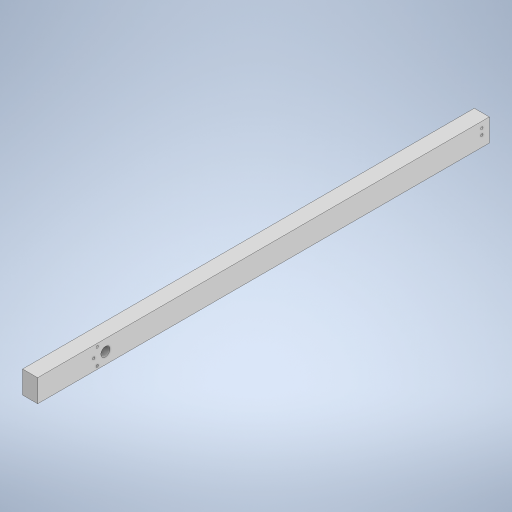
# Autodesk Inventor part: 射出_腕_真
Saved by Autodesk Inventor 2023 (Build 270158000, 158)
## iProperties
Created: 2022-04-27
Part Number: 射出_腕_真
Material: 一般
Document SubType Name: Modeling
Designer: yuta
Density: 1 g/cm^3
Appearance: 既定
Author: yuta
Autodesk Inventor part; units mm, degrees
ref_plane "YZ Plane" through (0, 0, 0) normal (1, 0, 0) x (0, 1, 0)
ref_plane "XZ Plane" through (0, 0, 0) normal (0, 1, 0) x (-1, 0, 0)
ref_plane "XY Plane" through (0, 0, 0) normal (0, 0, 1) x (1, 0, 0)
sketch "スケッチ1" plane through (0, 0, 0) normal (0, 0, 1) x (1, 0, 0)
  line L0 (0, 0) -> (20, 0)
  line L1 (20, 0) -> (20, 30)
  line L2 (20, 30) -> (0, 30)
  line L3 (0, 30) -> (0, 0)
  dimension "d0" = 20
  dimension "d1" = 30
  constraints: 8 end point, 2 parallel, 1 horizontal, 1 perpendicular
  measures "d0" distance of L2.end L1.end
  measures "d1" distance of L1.end L0.end
extrude "押し出し1" add sketch "スケッチ1" along normal blind 600
sketch "スケッチ2" plane through (20, 0, 0) normal (1, 0, 0) x (0, 0, -1)
  circle A0 centre (-510, 15) radius 6.05
  line L0 (0, 30) -> (-600, 30) projected
  line L1 (-600, 0) -> (-600, 30) projected
  point P0 (0, 0)
  dimension "d4" = 12.1
  dimension "d5" = 15
  dimension "d6" = 90
  constraints: 1 centre point
  measures "d4" diameter of A0
  measures "d5" distance from line of L0 A0.centre
  measures "d6" distance from line of L1 A0.centre
extrude "押し出し2" cut sketch "スケッチ2" against normal blind 600
sketch "スケッチ3" plane through (20, 0, 0) normal (1, 0, 0) x (0, 0, -1)
  line L0 (0, 30) -> (-600, 30) projected
  line L1 (0, 0) -> (0, 30) projected
  point P0 (-10, 22)
  point P1 (-10, 14)
  dimension "d9" = 8
  dimension "d10" = 10
  dimension "d11" = 8
  dimension "d12" = 10
  measures "d9" distance from line of L0 point (-10, 22)
  measures "d10" distance from line of L1 point (-10, 22)
  measures "d11" distance of point (-10, 22) point (-10, 14)
  measures "d12" distance from line of L1 point (-10, 14)
hole "穴1" at (20, 22, 10) at (20, 14, 10) direction (-1, 0, 0) diameter 3.2 end through all
sketch "スケッチ4" plane through (20, 0, 0) normal (1, 0, 0) x (0, 0, -1)
  circle A0 centre (-510, 15) radius 6.05 projected
  circle A1 centre (-510, 15) radius 15.5 construction
  line L0 (-510, 15) -> (-527.6598, 32.6598) construction
  line L1 (-510, 15) -> (-485.0253, 15) construction
  line L2 (-527.6598, 32.6598) -> (-527.6598, -10.8806) construction
  line L3 (0, 0) -> (-600, 0) projected
  line L4 (-510, 15) -> (-525.5285, -0.5285) construction
  line L5 (-510, 15) -> (-488.0394, 15) construction
  line L6 (-525.5285, -0.5285) -> (-520.9602, 4.0398)
  point P0 (-525.5, 15)
  point P1 (-520.9602, 25.9602)
  dimension "d20" = 31
  dimension "d21" = 135
  dimension "d22" = 135
  constraints: 12 end point, 3 point on circle, 2 coincident, 2 equal length, 2 horizontal, 2 point on line, 1 centre point, 1 perpendicular
  measures "d20" diameter of A1
  measures "d21" angle of L1 L0
  measures "d22" angle of L4 L5
hole "穴2" at (20, 15, 525.5) at (20, 25.9602, 520.9602) at (20, 4.0398, 520.9602) direction (-1, 0, 0) diameter 3.2 end through all
